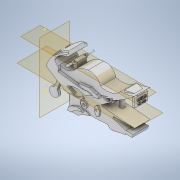
# Autodesk Inventor part: BMW S1000RR x Suzuki GXR R1000R
Saved by Autodesk Inventor 2021.1 (Build 251245000, 245)
## iProperties
Created: 2021-06-11
Part Number: BMW S1000RR x Suzuki GXR R1000R
Material: Generic
Document SubType Name: Modeling
Designer: as000166
Density: 1 g/cm^3
Appearance: Default
Author: as000166
Autodesk Inventor part; units mm, degrees
ref_plane "XY Plane" through (0, 0, 0) normal (0, 0, 1) x (1, 0, 0)
sketch "Sketch1" plane through (0, 0, 0) normal (0, 0, 1) x (1, 0, 0)
  point P0 (0, 0)
sketch "Sketch2" plane through (0, 0, 0) normal (0, 0, 1) x (1, 0, 0)
  line L0 (0, 119) -> (158.75, 119) construction
  line L1 (158.75, 119) -> (158.75, -0.0625) construction
  line L2 (158.75, -0.0625) -> (0, -0.0625) construction
  line L3 (0, -0.0625) -> (0, 119) construction
  arc A0 (51, 81) -> (25, 53) centre (68.8378, 38.3649) ccw
  arc A1 (25, 53) -> (53, 36) centre (68.2455, 92.669) ccw
  line L4 (53, 36) -> (61, 39)
  line L5 (61, 39) -> (51, 44)
  arc A2 (66, 47) -> (51, 44) centre (60.5, 35.5) ccw
  line L6 (66, 47) -> (75, 45)
  line L7 (51, 81) -> (52, 76)
  arc A3 (52, 76) -> (36, 65) centre (52.6429, 57.9286) ccw
  arc A4 (36, 65) -> (40, 60) centre (39.5, 63.7) ccw
  arc A5 (92, 62) -> (76, 72) centre (78.5, 58.2) ccw
  arc A6 (76, 72) -> (58, 63) centre (79.5, 42.5) ccw
  arc A7 (108.4973, 56.8115) -> (75, 45) centre (147.6347, -107.5867) ccw
  line L8 (108.4973, 56.8115) -> (107, 53.7361)
  arc A8 (107, 53.7361) -> (136, 72.8296) centre (44.0369, 180.937) ccw
  arc A9 (92, 62) -> (118, 69) centre (99.75, 85) ccw
  arc A10 (118, 69) -> (136, 72.8296) centre (117.9208, 113.5891) ccw
  arc A11 (40, 60) -> (58, 63) centre (47, 73.5) ccw
  point P0 (0, 0)
  constraints: 24 point on circle, 12 centre point, 10 end point, 2 other
extrude "Extrusion1" add sketch "Sketch2" along normal blind 20
sketch "Sketch3" plane through (0, 0, 20) normal (0, 0, 1) x (1, 0, 0)
  line L0 (0, 119) -> (158.75, 119) construction
  line L1 (158.75, 119) -> (158.75, -0.0625) construction
  line L2 (158.75, -0.0625) -> (0, -0.0625) construction
  line L3 (0, -0.0625) -> (0, 119) construction
  line L4 (53, 36) -> (61, 39) projected
  line L5 (55.6667, 37) -> (61, 35)
  arc A0 (61, 35) -> (69, 40) centre (60.0129, 45.4793) ccw
  arc A1 (72, 38) -> (69, 40) centre (69.1633, 36.9949) ccw
  arc A2 (72, 38) -> (75, 26) centre (73.8333, 32.0833) ccw
  arc A3 (51, 16) -> (53, 36) centre (9.8249, 30.2175) ccw
  line L6 (51, 16) -> (64, 16)
  arc A4 (79.375, 23) -> (64, 16) centre (91.4148, -23.8295) ccw
  line L7 (75, 26) -> (79.375, 23)
  point P0 (0, 0)
  constraints: 10 point on circle, 6 end point, 5 centre point, 1 point on line, 2 other
extrude "Extrusion2" add sketch "Sketch3" against normal blind 20
sketch "Sketch4" plane through (0, 0, 20) normal (0, 0, 1) x (1, 0, 0)
  line L0 (0.3227, 119.0807) -> (159.0727, 119.0807) construction
  line L1 (159.0727, 119.0807) -> (159.0727, 0.0182) construction
  line L2 (159.0727, 0.0182) -> (0.3227, 0.0182) construction
  line L3 (0.3227, 0.0182) -> (0.3227, 119.0807) construction
  line L4 (61, 39) -> (51, 44) projected
  line L5 (61, 39) -> (51.7187, 43.6406)
  arc A0 (74, 45) -> (51.7187, 43.6406) centre (64.1037, 23.9241) ccw
  arc A1 (88, 49) -> (74, 45) centre (89.4856, 17.3005) ccw
  line L6 (61, 39) -> (56.3594, 36.7402)
  line L7 (61, 35) -> (55.6667, 37) projected
  line L8 (56.3594, 36.7402) -> (61, 35)
  arc A2 (61, 35) -> (69, 40) centre (60.0129, 45.4793) ccw projected
  arc A3 (72, 38) -> (69, 40) centre (69.1633, 36.9949) ccw projected
  arc A4 (61, 35) -> (69, 40) centre (60.0129, 45.4793) ccw
  arc A5 (72, 38) -> (75, 26) centre (73.8333, 32.0833) ccw projected
  arc A6 (72, 38) -> (75, 26) centre (73.8333, 32.0833) ccw
  line L9 (75, 26) -> (79.6977, 23)
  arc A7 (109, 57) -> (88, 49) centre (124.1404, -14.3059) ccw
  line L10 (95, 51) -> (104.2405, 54.3798)
  line L11 (104.2405, 54.3798) -> (104.2405, 51)
  line L12 (104.2405, 51) -> (100.8487, 49.3312)
  line L13 (100.8487, 49.3312) -> (95, 51)
  line L14 (109, 57) -> (109, 56)
  line L15 (109, 56) -> (105, 55)
  line L16 (105, 55) -> (105, 51.3737)
  line L17 (105, 51.3737) -> (108, 53.1868)
  arc A8 (108, 53.1868) -> (111, 54) centre (108.9291, 55.6997) ccw
  line L18 (111, 54) -> (108, 51)
  line L19 (108, 51) -> (106, 51)
  line L20 (106, 51) -> (93, 42)
  line L21 (93, 42) -> (94, 40.5556)
  line L22 (94, 40.5556) -> (136, 36.9949)
  line L23 (136, 36.9949) -> (109, 36.7402)
  line L24 (109, 36.7402) -> (108, 34.2222)
  line L25 (108, 34.2222) -> (124.8199, 29)
  line L26 (124.8199, 29) -> (134, 29.0866)
  line L27 (134, 29.0866) -> (132.7312, 25)
  line L28 (132.7312, 25) -> (124.0566, 24.9182)
  line L29 (124.0566, 24.9182) -> (123.5572, 23.6607)
  line L30 (123.5572, 23.6607) -> (121.7595, 23.6438)
  line L31 (121.7595, 23.6438) -> (108, 20.3333)
  arc A9 (101.4448, 24.2894) -> (108, 20.3333) centre (106.8628, 25.8579) ccw
  arc A10 (79.6977, 23) -> (101.4448, 24.2894) centre (82.1967, 164.8855) ccw
  point P0 (0, 0)
  point P1 (110.6288, 53.6288)
  constraints: 52 end point, 16 point on circle, 8 centre point, 4 parallel, 3 point on line, 1 collinear, 1 concentric, 1 perpendicular, 1 vertical, 2 other
extrude "Extrusion3" add sketch "Sketch4" against normal blind 20 contours L4 A0 A1 A7 L14 L15 L16 L17 A8 L18 L19 L20 L21 L22 L23 L24 L25 L26 L27 L28 L29 L30 L31 A9 A10 L9 A5 A3 A2 L7 L6
sketch "Sketch5" plane through (0, 0, 20) normal (0, 0, 1) x (1, 0, 0)
  line L0 (0, 119) -> (158.75, 119) construction
  line L1 (158.75, 119) -> (158.75, -0.0625) construction
  line L2 (158.75, -0.0625) -> (0, -0.0625) construction
  line L3 (0, -0.0625) -> (0, 119) construction
  arc A0 (25, 53) -> (53, 36) centre (68.2455, 92.669) ccw projected
  line L4 (38.4827, 42.0925) -> (38.4827, 42.0925)
  line L5 (36.9918, 43) -> (32.2278, 31.5476)
  line L6 (40.4226, 41) -> (36, 30)
  arc A1 (32.2278, 31.5476) -> (36, 30) centre (32, 25.6214) ccw
  point P0 (0, 0)
  constraints: 6 end point, 6 point on circle, 1 centre point, 1 tangent, 2 other
extrude "Extrusion4" add sketch "Sketch5" against normal blind 20
sketch "Sketch6" plane through (0, 0, 20) normal (0, 0, 1) x (1, 0, 0)
  line L0 (0, 119) -> (158.75, 119) construction
  line L1 (158.75, 119) -> (158.75, -0.0625) construction
  line L2 (158.75, -0.0625) -> (0, -0.0625) construction
  line L3 (0, -0.0625) -> (0, 119) construction
  line L4 (52, 76) -> (51, 81) projected
  arc A0 (51, 81) -> (25, 53) centre (68.8378, 38.3649) ccw projected
  arc A1 (51.5, 78.5) -> (25, 53) centre (61.7966, 41.28) ccw
  arc A2 (51, 16) -> (53, 36) centre (9.8249, 30.2175) ccw projected
  arc A3 (25, 53) -> (53, 36) centre (128.25, 191.5) ccw
  line L5 (53, 36) -> (60.7223, 38.8959)
  line L6 (55.6667, 37) -> (61, 39) projected
  arc A4 (65.6621, 47.1556) -> (51.7187, 43.6406) centre (64.1037, 23.9241) ccw projected
  line L7 (61, 39) -> (51.7187, 43.6406)
  line L8 (51.7187, 43.6406) -> (51, 44) projected
  arc A5 (65.6621, 47.1556) -> (51.7187, 43.6406) centre (64.1037, 23.9241) ccw
  line L9 (65.6621, 47.1556) -> (75, 45)
  line L10 (75, 45) -> (84.0807, 49)
  arc A6 (101.5471, 55) -> (82, 48.1393) centre (147.6347, -107.5867) ccw projected
  line L11 (84.0807, 49) -> (77, 51)
  arc A7 (71.2365, 50) -> (77, 51) centre (72.017, 62.6105) ccw
  line L12 (71.2365, 50) -> (40, 54)
  line L13 (51.5, 78.5) -> (52, 76)
  arc A8 (52, 76) -> (36.049, 65) centre (52.301, 58.4983) ccw
  arc A9 (36.049, 65) -> (40, 60) centre (49.8238, 71.8238) ccw
  arc A10 (40, 54) -> (40, 60) centre (36, 57) ccw
  point P0 (0, 0)
  point P1 (27.4841, 59)
  constraints: 15 point on circle, 14 end point, 7 centre point, 1 collinear, 1 concentric, 1 midpoint, 1 point on line, 2 other
extrude "Extrusion5" add sketch "Sketch6" along normal blind 3 and the other way blind 23 contours A8 A9 A10 L12 A7 L11 L10 L9 A4 L7 L6 L5 A3 A0 A1 L4
sketch "Sketch7" plane through (36.9918, 43, 0) normal (-0.9233002, 0.3840791, 0) x (0, 0, 1)
  line L0 (0, -0.3147) -> (20, -0.3147) projected
  line L1 (4, -0.3147) -> (17, -0.3147)
  line L2 (17, -0.3147) -> (17, -23.8935)
  line L3 (20, -23.8935) -> (0, -23.8935) projected
  line L4 (17, -23.8935) -> (4, -23.8935)
  line L5 (4, -23.8935) -> (4, -0.3147)
  point P0 (0, -53.9097)
  constraints: 8 end point, 3 point on line, 2 perpendicular, 1 horizontal
extrude "Extrusion6" cut sketch "Sketch7" along normal blind 9 and the other way blind 9
sketch "Sketch10" plane through (0, 0, 20) normal (0, 0, 1) x (1, 0, 0)
  line L0 (0, 117) -> (158.75, 117) construction
  line L1 (158.75, 117) -> (158.75, -2.0625) construction
  line L2 (158.75, -2.0625) -> (0, -2.0625) construction
  line L3 (0, -2.0625) -> (0, 117) construction
  line L4 (66, 54) -> (81, 56)
  arc A0 (81, 56) -> (90.0213, 52.996) centre (96.5, 87.5) ccw
  arc A1 (93, 49.9999) -> (90.0213, 52.996) centre (89.3337, 49.3336) ccw
  arc A2 (66, 54) -> (75.4151, 50.8696) centre (73.5, 60.8333) ccw
  arc A3 (84.2663, 49.9712) -> (75.4151, 50.8696) centre (78.3411, 35.6463) ccw
  line L5 (84.2663, 49.9712) -> (86, 48)
  line L6 (86, 48) -> (93, 49.9999)
  point P0 (0, 0)
  constraints: 8 point on circle, 6 end point, 4 centre point, 2 tangent, 2 other
extrude "Extrusion7" add sketch "Sketch10" along normal blind 3 and the other way blind 23
ref_plane "Work Plane1" through (0, 70, 0) normal (0, 1, 0) x (-1, 0, 0)
sketch "Sketch11" plane through (0, 70, 0) normal (0, 1, 0) x (-1, 0, 0)
  line L0 (-53, 0) -> (-53, 20) projected
  line L1 (-53, 16) -> (-53, 4)
  line L2 (-53, 4) -> (-58, 4)
  line L3 (-58, 4) -> (-58, 16)
  line L4 (-58, 0) -> (-58, 20) projected
  line L5 (-53, 16) -> (-58, 16)
  point P0 (0, 0)
  dimension "d27" = 12
  dimension "d28" = 5
  constraints: 8 end point, 3 point on line, 1 perpendicular
  measures "d27" distance of L1.start L1.end
  measures "d28" distance of L1.end L2.end
extrude "Extrusion8" add sketch "Sketch11" against normal up to surface
sketch "Sketch12" plane through (0, 70, 0) normal (0, 1, 0) x (1, 0, 0)
  point P0 (0, 0)
sketch "Sketch13" plane through (0, 70, 0) normal (0, 1, 0) x (1, 0, 0)
  line L0 (53, -4) -> (53, -16) projected
  line L1 (53, -4) -> (53, -16)
  line L2 (53, -16) -> (60.2469, -16) construction
  line L3 (58, -16) -> (58, -20) projected
  line L4 (58, -16) -> (58, -4)
  line L5 (58, -4) -> (58, -16)
  line L6 (58, 0) -> (58, -4) projected
  line L7 (58, -4) -> (58, -16)
  line L8 (53, -16) -> (54, -20)
  line L9 (54, -20) -> (56, -20)
  line L10 (58, -20) -> (40, -20) projected
  line L11 (58, -16) -> (56, -20)
  line L12 (53, -4) -> (54, 0)
  line L13 (58, 0) -> (40, 0) projected
  line L14 (54, 0) -> (56, 0)
  line L15 (58, -4) -> (56, 0)
  line L16 (54, -16) -> (57, -16)
  line L17 (57, -16) -> (56, -18)
  line L18 (56, -18) -> (54.5, -18)
  line L19 (54.5, -18) -> (54, -16)
  line L20 (54, -4) -> (56.8824, -4)
  line L21 (56, -2) -> (54.5, -2)
  line L22 (54.5, -2) -> (54, -4)
  line L23 (56.8824, -4) -> (56, -2)
  point P0 (0, 0)
  dimension "d31" = 12
  dimension "d35" = 1.5
  dimension "d36" = 1.5
  constraints: 38 end point, 5 point on line, 3 collinear, 2 horizontal, 1 parallel, 1 vertical
  measures "d31" distance of L0.start L0.end
  measures "d35" distance of L17.end L18.end
  measures "d36" distance of L21.start L21.end
extrude "Extrusion9" add sketch "Sketch13" against normal blind 2 contours L12 L13 L15 L4 L11 L9 L8 L0
sketch "Sketch14" plane through (54, 70, 20) normal (0, 0, 1) x (1, 0, 0)
  circle A0 centre (1, -1) radius 1
  point P0 (-54, -70)
  constraints: 1 centre point
extrude "Extrusion10" add sketch "Sketch14" along normal blind 7
sketch "Sketch15" plane through (56, 70, 0) normal (0, 0, -1) x (-1, 0, 0)
  circle A0 centre (1, -1) radius 1
  line L0 (2, 0) -> (2, -1) projected
  point P0 (56, -70)
  constraints: 1 horizontal alignment, 1 vertical, 1 other
extrude "Extrusion11" add sketch "Sketch15" along normal blind 8
sketch "Sketch16" plane through (0, 70, 0) normal (0, 1, 0) x (-1, 0, 0)
  line L0 (-121, 18) -> (-121, 2)
  line L1 (-121, 2) -> (-134, 5.4833)
  line L2 (-134, 20) -> (-134, 0) projected
  line L3 (-121, 18) -> (-108.0418, 18) construction
  line L4 (-121, 18) -> (-134, 14.5167)
  line L5 (-121, 18) -> (-107.5414, 18) construction
  line L6 (-134, 14.5167) -> (-134, 5.4833)
  point P0 (0, 0)
  dimension "d43" = 75
  dimension "d45" = 165
  constraints: 12 end point, 2 horizontal, 2 point on line, 1 collinear, 1 equal length, 1 vertical
  measures "d43" angle of L0 L1
  measures "d45" angle of L4 L5
extrude "Extrusion12" add sketch "Sketch16" along normal blind 1 and the other way blind 0.95
sketch "Sketch17" plane through (134, 69.05, 5.4833) normal (1, 0, 0) x (0, 0, -1)
  line L0 (3.4833, 1.95) -> (-12.5167, 1.95) projected
  line L1 (-9, 1.95) -> (0, 1.95)
  line L2 (0, 1.95) -> (0, -0.05)
  line L3 (5.4833, -0.05) -> (-14.5167, -0.05) projected
  line L4 (0, -0.05) -> (4, -0.05)
  line L5 (-9.0333, 0) -> (-9.0333, 1.95) projected
  line L6 (-9.0333, 0) -> (-13.0333, 0)
  line L7 (-13.0333, 0) -> (-13.0333, -5)
  line L8 (-13.0333, -5) -> (-13.0333, -11)
  line L9 (4, -0.05) -> (4, -11)
  line L10 (-13.0333, -11) -> (4, -11)
  point P0 (5.4833, -69.05)
  point P1 (-13.0333, -0.05)
  dimension "d51" = 4
  dimension "d52" = 5
  dimension "d75" = 6
  constraints: 16 end point, 3 point on line, 2 perpendicular, 1 horizontal, 1 vertical
  measures "d51" distance of L5.start L6.end
  measures "d52" distance of L6.end L7.end
  measures "d75" distance of L7.end L8.end
extrude "Extrusion13" add sketch "Sketch17" along normal blind 0.75 and the other way blind 2 contours L3 L9 L10 L8 L7
sketch "Sketch18" plane through (0, 0, 20) normal (0, 0, 1) x (1, 0, 0)
  line L0 (0, 118) -> (158.75, 118) construction
  line L1 (158.75, 118) -> (158.75, -1.0625) construction
  line L2 (158.75, -1.0625) -> (0, -1.0625) construction
  line L3 (0, -1.0625) -> (0, 118) construction
  arc A0 (72, 24) -> (57, 17) centre (72.2778, 3.8333) ccw
  line L4 (57, 17) -> (52, 17)
  arc A1 (59, 25) -> (52, 17) centre (65.1, 12.6) ccw
  line L5 (59, 25) -> (65, 27)
  arc A2 (72, 24) -> (65, 27) centre (64.5774, 16.3472) ccw
  point P0 (0, 0)
  constraints: 6 point on circle, 4 end point, 3 centre point, 2 other
extrude "Extrusion14" add sketch "Sketch18" along normal blind 3 and the other way blind 23
sketch "Sketch19" plane through (0, 0, 20) normal (0, 0, 1) x (1, 0, 0)
  line L0 (0, 119) -> (158.75, 119) construction
  line L1 (158.75, 119) -> (158.75, -0.0625) construction
  line L2 (158.75, -0.0625) -> (0, -0.0625) construction
  line L3 (0, -0.0625) -> (0, 119) construction
  circle A0 centre (72, 32) radius 4
  circle A1 centre (72, 32) radius 1.7911
  point P0 (0, 0)
  constraints: 2 centre point, 1 coincident, 2 other
extrude "Extrusion15" add sketch "Sketch19" along normal blind 1.5 and the other way blind 21.5
sketch "Sketch20" plane through (0, 0, 20) normal (0, 0, 1) x (1, 0, 0)
  line L0 (0, 119) -> (158.75, 119) construction
  line L1 (158.75, 119) -> (158.75, -0.0625) construction
  line L2 (158.75, -0.0625) -> (0, -0.0625) construction
  line L3 (0, -0.0625) -> (0, 119) construction
  line L4 (87, 38) -> (90, 40)
  arc A0 (91, 28) -> (90, 40) centre (79.25, 33.0625) ccw
  arc A1 (87, 38) -> (88.5, 26.8549) centre (95.5979, 33.4837) ccw
  line L5 (88.5, 26.8549) -> (91, 28)
  circle A2 centre (88, 34) radius 1
  point P0 (0, 0)
  constraints: 4 end point, 4 point on circle, 3 centre point, 2 other
extrude "Extrusion16" add sketch "Sketch20" along normal blind 1.5 and the other way blind 21.5
sketch "Sketch21" plane through (134.75, 69.05, 5.4833) normal (1, 0, 0) x (0, 0, -1)
  line L0 (-10.1051, -1.0894) -> (0.9281, -1.0894) construction
  line L1 (0.9281, -1.0894) -> (0.9281, -4.0805) construction
  line L2 (0.9281, -4.0805) -> (-10.1051, -4.0805) construction
  line L3 (-10.1051, -4.0805) -> (-10.1051, -1.0894) construction
  line L4 (-8.5838, -2.0986) -> (-7.0277, -2.0986)
  line L5 (-7.0277, -2.0986) -> (-7.0277, -5.0947)
  line L6 (-7.0277, -5.0947) -> (-7.3562, -5.0947)
  line L7 (-7.3562, -5.0947) -> (-7.3562, -4.8823)
  line L8 (-7.3562, -4.8823) -> (-8.2553, -4.8823)
  line L9 (-8.2553, -4.8823) -> (-8.2553, -5.1935)
  line L10 (-8.2553, -5.1935) -> (-8.5838, -5.1935)
  line L11 (-8.5838, -5.1935) -> (-8.5838, -2.0986)
  line L12 (-10.582, -2.968) -> (-10.582, -2.6568)
  line L13 (-10.582, -2.6568) -> (-9.8114, -2.6568)
  line L14 (-9.8114, -2.6568) -> (-9.8114, -2.148)
  spline S0 degree 2 poles (-9.8114, -2.148) (-10.2214, -2.2146) (-10.4511, -2.2295) knots 0 0 0 1 1 1
  line L15 (-10.4511, -2.2295) -> (-10.582, -1.9355)
  spline S1 degree 2 poles (-10.582, -1.9355) (-9.7472, -1.854) (-9.0901, -1.607) knots 0 0 0 1 1 1
  line L16 (-9.0901, -1.607) -> (-8.895, -1.9034)
  spline S2 degree 2 poles (-8.895, -1.9034) (-8.8777, -2.017) (-8.9938, -1.9528) knots 0 0 0 1 1 1
  line L17 (-8.9938, -1.9528) -> (-9.4853, -2.0837)
  line L18 (-9.4853, -2.0837) -> (-9.4853, -2.6568)
  line L19 (-9.4853, -2.6568) -> (-8.7468, -2.6568)
  line L20 (-8.7468, -2.6568) -> (-8.7468, -2.968)
  line L21 (-8.7468, -2.968) -> (-9.4853, -2.968)
  line L22 (-9.4853, -2.968) -> (-9.4853, -3.3113)
  spline S3 degree 2 poles (-9.4853, -3.3113) (-8.9938, -3.5238) (-8.732, -3.835) knots 0 0 0 1 1 1
  line L23 (-8.732, -3.835) -> (-8.9444, -4.1462)
  spline S4 degree 2 poles (-8.9444, -4.1462) (-9.2383, -3.8177) (-9.4853, -3.6547) knots 0 0 0 1 1 1
  line L24 (-9.4853, -3.6547) -> (-9.4853, -5.275)
  line L25 (-9.4853, -5.275) -> (-9.8114, -5.275)
  line L26 (-9.8114, -5.275) -> (-9.8114, -3.7041)
  spline S5 degree 2 poles (-9.8114, -3.7041) (-10.0584, -4.1956) (-10.4338, -4.571) knots 0 0 0 1 1 1
  line L27 (-10.4338, -4.571) -> (-10.6783, -4.2771)
  spline S6 degree 2 poles (-10.6783, -4.2771) (-10.0732, -3.7041) (-9.8287, -2.968) knots 0 0 0 1 1 1
  line L28 (-9.8287, -2.968) -> (-10.582, -2.968)
  line L29 (-8.2553, -2.4098) -> (-8.2553, -4.571)
  line L30 (-8.2553, -4.571) -> (-7.3562, -4.571)
  line L31 (-7.3562, -4.571) -> (-7.3562, -2.4098)
  line L32 (-7.3562, -2.4098) -> (-8.2553, -2.4098)
  spline S7 degree 2 poles (-3.6882, -4.0474) (-3.8833, -4.7341) (-4.5058, -5.275) knots 0 0 0 1 1 1
  line L33 (-4.5058, -5.275) -> (-4.7207, -4.9638)
  spline S8 degree 2 poles (-4.7207, -4.9638) (-3.8833, -4.3265) (-3.8833, -3.3928) knots 0 0 0 1 1 1
  line L34 (-3.8833, -3.3928) -> (-3.8833, -2.558)
  line L35 (-3.8833, -2.558) -> (-4.0315, -2.558)
  spline S9 degree 2 poles (-4.0315, -2.558) (-4.0982, -2.8025) (-4.3255, -3.2125) knots 0 0 0 1 1 1
  line L36 (-4.3255, -3.2125) -> (-4.6046, -3.0643)
  spline S10 degree 2 poles (-4.6046, -3.0643) (-4.2291, -2.5259) (-4.1303, -1.5922) knots 0 0 0 1 1 1
  line L37 (-4.1303, -1.5922) -> (-3.8191, -1.6416)
  spline S11 degree 2 poles (-3.8191, -1.6416) (-3.7203, -1.6564) (-3.8364, -1.7379) knots 0 0 0 1 1 1
  spline S12 degree 2 poles (-3.8364, -1.7379) (-3.9327, -2.1652) (-3.9673, -2.2962) knots 0 0 0 1 1 1
  line L38 (-3.9673, -2.2962) -> (-3.0658, -2.2962)
  line L39 (-3.0658, -2.2962) -> (-3.0336, -2.2146)
  line L40 (-3.0336, -2.2146) -> (-2.7224, -2.4098)
  spline S13 degree 2 poles (-2.7224, -2.4098) (-2.673, -2.4419) (-2.7545, -2.4913) knots 0 0 0 1 1 1
  spline S14 degree 2 poles (-2.7545, -2.4913) (-2.8854, -3.0816) (-3.1152, -3.541) knots 0 0 0 1 1 1
  line L41 (-3.1152, -3.541) -> (-3.3943, -3.425)
  spline S15 degree 2 poles (-3.3943, -3.425) (-3.1646, -2.968) (-3.083, -2.558) knots 0 0 0 1 1 1
  line L42 (-3.083, -2.558) -> (-3.5573, -2.558)
  line L43 (-3.5573, -2.558) -> (-3.5573, -3.3434)
  spline S16 degree 2 poles (-3.5573, -3.3434) (-3.5573, -4.2771) (-2.7051, -4.9317) knots 0 0 0 1 1 1
  line L44 (-2.7051, -4.9317) -> (-2.9521, -5.2108)
  spline S17 degree 2 poles (-2.9521, -5.2108) (-3.5252, -4.6871) (-3.6882, -4.0474) knots 0 0 0 1 1 1
  spline S18 degree 2 poles (-4.7528, -5.0132) (-4.7528, -5.2602) (-4.9973, -5.2602) knots 0 0 0 1 1 1
  line L45 (-4.9973, -5.2602) -> (-5.4073, -5.2602)
  line L46 (-5.4073, -5.2602) -> (-5.4567, -4.949)
  line L47 (-5.4567, -4.949) -> (-5.0961, -4.949)
  spline S19 degree 2 poles (-5.0961, -4.949) (-5.0294, -4.949) (-5.0294, -4.8823) knots 0 0 0 1 1 1
  line L48 (-5.0294, -4.8823) -> (-5.0294, -3.7041)
  line L49 (-5.0294, -3.7041) -> (-6.4719, -3.7041)
  line L50 (-6.4719, -3.7041) -> (-6.4719, -3.3928)
  line L51 (-6.4719, -3.3928) -> (-4.4416, -3.3928)
  line L52 (-4.4416, -3.3928) -> (-4.4416, -3.7041)
  line L53 (-4.4416, -3.7041) -> (-4.7528, -3.7041)
  line L54 (-4.7528, -3.7041) -> (-4.7528, -5.0132)
  spline S20 degree 2 poles (-4.7528, -3.0149) (-4.7528, -3.2768) (-4.9652, -3.2768) knots 0 0 0 1 1 1
  line L55 (-4.9652, -3.2768) -> (-5.2443, -3.2768)
  line L56 (-5.2443, -3.2768) -> (-5.2764, -3.0149)
  line L57 (-5.2764, -3.0149) -> (-5.0961, -3.0149)
  spline S21 degree 2 poles (-5.0961, -3.0149) (-5.0294, -3.0149) (-5.0294, -2.9507) knots 0 0 0 1 1 1
  line L58 (-5.0294, -2.9507) -> (-5.0294, -2.017)
  line L59 (-5.0294, -2.017) -> (-6.3558, -2.017)
  line L60 (-6.3558, -2.017) -> (-6.3558, -1.7058)
  line L61 (-6.3558, -1.7058) -> (-4.4564, -1.7058)
  line L62 (-4.4564, -1.7058) -> (-4.4564, -2.017)
  line L63 (-4.4564, -2.017) -> (-4.7528, -2.017)
  line L64 (-4.7528, -2.017) -> (-4.7528, -3.0149)
  line L65 (-5.2937, -3.8992) -> (-5.2937, -4.702)
  line L66 (-5.2937, -4.702) -> (-5.9804, -4.702)
  line L67 (-5.9804, -4.702) -> (-5.9804, -4.8823)
  line L68 (-5.9804, -4.8823) -> (-6.2101, -4.8823)
  line L69 (-6.2101, -4.8823) -> (-6.2101, -3.8992)
  line L70 (-6.2101, -3.8992) -> (-5.2937, -3.8992)
  line L71 (-5.3085, -2.2146) -> (-5.3085, -2.9507)
  line L72 (-5.3085, -2.9507) -> (-5.931, -2.9507)
  line L73 (-5.931, -2.9507) -> (-5.931, -3.0989)
  line L74 (-5.931, -3.0989) -> (-6.1607, -3.0989)
  line L75 (-6.1607, -3.0989) -> (-6.1607, -2.2146)
  line L76 (-6.1607, -2.2146) -> (-5.3085, -2.2146)
  line L77 (-5.521, -4.0968) -> (-5.9804, -4.0968)
  line L78 (-5.9804, -4.0968) -> (-5.9804, -4.5068)
  line L79 (-5.9804, -4.5068) -> (-5.521, -4.5068)
  line L80 (-5.521, -4.5068) -> (-5.521, -4.0968)
  line L81 (-5.5382, -2.4098) -> (-5.931, -2.4098)
  line L82 (-5.931, -2.4098) -> (-5.931, -2.7531)
  line L83 (-5.931, -2.7531) -> (-5.5382, -2.7531)
  line L84 (-5.5382, -2.7531) -> (-5.5382, -2.4098)
  spline S22 degree 2 poles (1.2247, -2.3604) (1.3877, -2.395) (1.2395, -2.4913) knots 0 0 0 1 1 1
  line L85 (1.2395, -2.4913) -> (1.2395, -5.112)
  line L86 (1.2395, -5.112) -> (0.864, -5.112)
  line L87 (0.864, -5.112) -> (0.864, -4.8502)
  line L88 (0.864, -4.8502) -> (-1.6406, -4.8502)
  line L89 (-1.6406, -4.8502) -> (-1.6406, -5.1762)
  line L90 (-1.6406, -5.1762) -> (-2.0185, -5.1762)
  line L91 (-2.0185, -5.1762) -> (-2.0185, -2.3604)
  line L92 (-2.0185, -2.3604) -> (-1.6578, -2.3604)
  spline S23 degree 2 poles (-1.6578, -2.3604) (-1.4948, -2.395) (-1.6406, -2.4913) knots 0 0 0 1 1 1
  line L93 (-1.6406, -2.4913) -> (-1.6406, -4.4895)
  line L94 (-1.6406, -4.4895) -> (-0.5933, -4.4895)
  line L95 (-0.5933, -4.4895) -> (-0.5933, -1.6737)
  line L96 (-0.5933, -1.6737) -> (-0.2326, -1.6737)
  spline S24 degree 2 poles (-0.2326, -1.6737) (-0.0696, -1.7058) (-0.2178, -1.8046) knots 0 0 0 1 1 1
  line L97 (-0.2178, -1.8046) -> (-0.2178, -4.4895)
  line L98 (-0.2178, -4.4895) -> (0.864, -4.4895)
  line L99 (0.864, -4.4895) -> (0.864, -2.3604)
  line L100 (0.864, -2.3604) -> (1.2247, -2.3604)
  line L101 (-7.7403, -8.9028) -> (-8.1034, -8.9028)
  line L102 (-8.1034, -8.9028) -> (-8.1034, -9.9501)
  line L103 (-8.1034, -9.9501) -> (-8.4961, -9.9501)
  line L104 (-8.4961, -9.9501) -> (-8.4961, -8.9028)
  line L105 (-8.4961, -8.9028) -> (-9.8422, -8.9028)
  line L106 (-9.8422, -8.9028) -> (-9.8422, -8.473)
  line L107 (-9.8422, -8.473) -> (-8.4788, -6.9021)
  line L108 (-8.4788, -6.9021) -> (-8.1034, -6.9021)
  line L109 (-8.1034, -6.9021) -> (-8.1034, -8.5743)
  line L110 (-8.1034, -8.5743) -> (-7.7403, -8.5743)
  line L111 (-7.7403, -8.5743) -> (-7.7403, -8.9028)
  line L112 (-8.4961, -8.5743) -> (-8.4961, -7.3838)
  line L113 (-8.4961, -7.3838) -> (-9.5211, -8.5743)
  line L114 (-9.5211, -8.5743) -> (-8.4961, -8.5743)
  line L115 (-5.5345, -9.9501) -> (-7.4142, -9.9501)
  line L116 (-7.4142, -9.9501) -> (-7.4142, -9.5179)
  spline S25 degree 2 poles (-7.4142, -9.5179) (-7.2117, -9.3277) (-6.8511, -8.9745) (-6.6782, -8.7843) knots 0 0 0 1 2 2 2
  spline S26 degree 2 poles (-6.6782, -8.7843) (-6.3299, -8.4014) (-6.0755, -7.942) (-6.0755, -7.6975) knots 0 0 0 1 2 2 2
  spline S27 degree 2 poles (-6.0755, -7.6975) (-6.0755, -7.569) (-6.1545, -7.3764) (-6.2261, -7.3146) knots 0 0 0 1 2 2 2
  spline S28 degree 2 poles (-6.2261, -7.3146) (-6.2978, -7.2529) (-6.4855, -7.1911) (-6.5991, -7.1911) knots 0 0 0 1 2 2 2
  spline S29 degree 2 poles (-6.5991, -7.1911) (-6.7078, -7.1911) (-6.9301, -7.2455) (-7.0314, -7.2874) knots 0 0 0 1 2 2 2
  spline S30 degree 2 poles (-7.0314, -7.2874) (-7.1178, -7.322) (-7.2784, -7.4208) (-7.3278, -7.4554) knots 0 0 0 1 2 2 2
  line L117 (-7.3278, -7.4554) -> (-7.35, -7.4554)
  line L118 (-7.35, -7.4554) -> (-7.35, -7.0207)
  spline S31 degree 2 poles (-7.35, -7.0207) (-7.224, -6.9589) (-6.772, -6.8379) (-6.5695, -6.8379) knots 0 0 0 1 2 2 2
  spline S32 degree 2 poles (-6.5695, -6.8379) (-6.1422, -6.8379) (-5.6605, -7.2899) (-5.6605, -7.6752) knots 0 0 0 1 2 2 2
  spline S33 degree 2 poles (-5.6605, -7.6752) (-5.6605, -7.8555) (-5.7445, -8.1569) (-5.8186, -8.2853) knots 0 0 0 1 2 2 2
  spline S34 degree 2 poles (-5.8186, -8.2853) (-5.8927, -8.4187) (-6.1076, -8.6805) (-6.2261, -8.8065) knots 0 0 0 1 2 2 2
  spline S35 degree 2 poles (-6.2261, -8.8065) (-6.4188, -9.0165) (-6.8906, -9.466) (-7.0314, -9.5969) knots 0 0 0 1 2 2 2
  line L119 (-7.0314, -9.5969) -> (-5.5345, -9.5969)
  line L120 (-5.5345, -9.5969) -> (-5.5345, -9.9501)
  line L121 (-4.0105, -8.8016) -> (-5.164, -8.8016)
  line L122 (-5.164, -8.8016) -> (-5.164, -8.4311)
  line L123 (-5.164, -8.4311) -> (-4.0105, -8.4311)
  line L124 (-4.0105, -8.4311) -> (-4.0105, -8.8016)
  spline S36 degree 2 poles (-1.6788, -8.9621) (-1.6788, -9.1968) (-1.8345, -9.5944) (-1.9654, -9.7278) knots 0 0 0 1 2 2 2
  spline S37 degree 2 poles (-1.9654, -9.7278) (-2.1012, -9.8686) (-2.4421, -10.0143) (-2.6471, -10.0143) knots 0 0 0 1 2 2 2
  spline S38 degree 2 poles (-2.6471, -10.0143) (-2.8521, -10.0143) (-3.1905, -9.876) (-3.3189, -9.7377) knots 0 0 0 1 2 2 2
  spline S39 degree 2 poles (-3.3189, -9.7377) (-3.477, -9.5722) (-3.6549, -9.0165) (-3.6549, -8.6114) knots 0 0 0 1 2 2 2
  spline S40 degree 2 poles (-3.6549, -8.6114) (-3.6549, -8.2137) (-3.4918, -7.574) (-3.3214, -7.3368) knots 0 0 0 1 2 2 2
  spline S41 degree 2 poles (-3.3214, -7.3368) (-3.1559, -7.1047) (-2.6323, -6.8453) (-2.2889, -6.8453) knots 0 0 0 1 2 2 2
  spline S42 degree 2 poles (-2.2889, -6.8453) (-2.1877, -6.8453) (-2.0098, -6.8651) (-1.9431, -6.8873) knots 0 0 0 1 2 2 2
  line L125 (-1.9431, -6.8873) -> (-1.9431, -7.28)
  line L126 (-1.9431, -7.28) -> (-1.9604, -7.28)
  spline S43 degree 2 poles (-1.9604, -7.28) (-2.0172, -7.2504) (-2.2247, -7.1985) (-2.3433, -7.1985) knots 0 0 0 1 2 2 2
  spline S44 degree 2 poles (-2.3433, -7.1985) (-2.7237, -7.1985) (-3.1905, -7.7123) (-3.235, -8.2162) knots 0 0 0 1 2 2 2
  spline S45 degree 2 poles (-3.235, -8.2162) (-3.0892, -8.1149) (-2.7829, -8.0037) (-2.6002, -8.0037) knots 0 0 0 1 2 2 2
  spline S46 degree 2 poles (-2.6002, -8.0037) (-2.4223, -8.0037) (-2.1556, -8.0754) (-2.0098, -8.1841) knots 0 0 0 1 2 2 2
  spline S47 degree 2 poles (-2.0098, -8.1841) (-1.8419, -8.31) (-1.6788, -8.7003) (-1.6788, -8.9621) knots 0 0 0 1 2 2 2
  spline S48 degree 2 poles (-2.0938, -8.9794) (-2.0938, -8.7917) (-2.1926, -8.5373) (-2.3013, -8.4483) knots 0 0 0 1 2 2 2
  spline S49 degree 2 poles (-2.3013, -8.4483) (-2.3828, -8.3841) (-2.5853, -8.3421) (-2.6915, -8.3421) knots 0 0 0 1 2 2 2
  spline S50 degree 2 poles (-2.6915, -8.3421) (-2.8348, -8.3421) (-3.104, -8.4286) (-3.235, -8.5101) knots 0 0 0 1 2 2 2
  spline S51 degree 2 poles (-3.235, -8.5101) (-3.2374, -8.5546) (-3.2424, -8.6385) (-3.2424, -8.7028) knots 0 0 0 1 2 2 2
  spline S52 degree 2 poles (-3.2424, -8.7028) (-3.2424, -9.0189) (-3.1189, -9.4067) (-3.025, -9.508) knots 0 0 0 1 2 2 2
  spline S53 degree 2 poles (-3.025, -9.508) (-2.9386, -9.6043) (-2.7508, -9.6809) (-2.6446, -9.6809) knots 0 0 0 1 2 2 2
  spline S54 degree 2 poles (-2.6446, -9.6809) (-2.3976, -9.6809) (-2.0938, -9.3301) (-2.0938, -8.9794) knots 0 0 0 1 2 2 2
  spline S55 degree 2 poles (-1.4022, -7.8926) (-1.4022, -7.6579) (-1.2491, -7.2677) (-1.1157, -7.1269) knots 0 0 0 1 2 2 2
  spline S56 degree 2 poles (-1.1157, -7.1269) (-0.9897, -6.991) (-0.6217, -6.8404) (-0.434, -6.8404) knots 0 0 0 1 2 2 2
  spline S57 degree 2 poles (-0.434, -6.8404) (-0.224, -6.8404) (0.1169, -6.9812) (0.2428, -7.1145) knots 0 0 0 1 2 2 2
  spline S58 degree 2 poles (0.2428, -7.1145) (0.4009, -7.2825) (0.5738, -7.8259) (0.5738, -8.2433) knots 0 0 0 1 2 2 2
  spline S59 degree 2 poles (0.5738, -8.2433) (0.5738, -8.6212) (0.4034, -9.298) (0.2379, -9.5228) knots 0 0 0 1 2 2 2
  spline S60 degree 2 poles (0.2379, -9.5228) (0.0625, -9.7599) (-0.4315, -10.0094) (-0.7921, -10.0094) knots 0 0 0 1 2 2 2
  spline S61 degree 2 poles (-0.7921, -10.0094) (-0.8736, -10.0094) (-1.0589, -9.9921) (-1.1379, -9.9674) knots 0 0 0 1 2 2 2
  line L127 (-1.1379, -9.9674) -> (-1.1379, -9.5747)
  line L128 (-1.1379, -9.5747) -> (-1.1181, -9.5747)
  spline S62 degree 2 poles (-1.1181, -9.5747) (-1.0663, -9.6043) (-0.8489, -9.6562) (-0.7378, -9.6562) knots 0 0 0 1 2 2 2
  spline S63 degree 2 poles (-0.7378, -9.6562) (-0.3376, -9.6562) (0.1193, -9.1276) (0.1514, -8.6385) knots 0 0 0 1 2 2 2
  spline S64 degree 2 poles (0.1514, -8.6385) (-0.0116, -8.7497) (-0.308, -8.851) (-0.4834, -8.851) knots 0 0 0 1 2 2 2
  spline S65 degree 2 poles (-0.4834, -8.851) (-0.6513, -8.851) (-0.9304, -8.7769) (-1.0712, -8.6707) knots 0 0 0 1 2 2 2
  spline S66 degree 2 poles (-1.0712, -8.6707) (-1.2342, -8.5447) (-1.4022, -8.1618) (-1.4022, -7.8926) knots 0 0 0 1 2 2 2
  spline S67 degree 2 poles (0.1613, -8.1519) (0.1613, -7.8432) (0.0477, -7.4529) (-0.0536, -7.3467) knots 0 0 0 1 2 2 2
  spline S68 degree 2 poles (-0.0536, -7.3467) (-0.1425, -7.2479) (-0.3277, -7.1738) (-0.4364, -7.1738) knots 0 0 0 1 2 2 2
  spline S69 degree 2 poles (-0.4364, -7.1738) (-0.6884, -7.1738) (-0.9872, -7.5344) (-0.9872, -7.8753) knots 0 0 0 1 2 2 2
  spline S70 degree 2 poles (-0.9872, -7.8753) (-0.9872, -8.068) (-0.8884, -8.3174) (-0.7798, -8.4064) knots 0 0 0 1 2 2 2
  spline S71 degree 2 poles (-0.7798, -8.4064) (-0.7007, -8.4706) (-0.5056, -8.5126) (-0.392, -8.5126) knots 0 0 0 1 2 2 2
  spline S72 degree 2 poles (-0.392, -8.5126) (-0.2611, -8.5126) (0.0403, -8.4212) (0.1539, -8.3446) knots 0 0 0 1 2 2 2
  spline S73 degree 2 poles (0.1539, -8.3446) (0.1564, -8.315) (0.1613, -8.2137) (0.1613, -8.1519) knots 0 0 0 1 2 2 2
  point P0 (5.4833, -69.05)
  constraints: 2 other
extrude "Extrusion17" add sketch "Sketch21" along normal blind 1
sketch "Sketch22" plane through (0, 69.05, 0) normal (0, -1, 0) x (1, 0, 0)
  point P0 (0, 0)
sketch "Sketch23" plane through (0, 0, 20) normal (0, 0, 1) x (1, 0, 0)
  line L0 (0, 119) -> (158.75, 119) construction
  line L1 (158.75, 119) -> (158.75, -0.0625) construction
  line L2 (158.75, -0.0625) -> (0, -0.0625) construction
  line L3 (0, -0.0625) -> (0, 119) construction
  arc A0 (51, 16) -> (53, 36) centre (9.8249, 30.2175) ccw projected
  line L4 (51, 16) -> (64, 16)
  arc A1 (79.375, 23) -> (64, 16) centre (91.4148, -23.8295) ccw projected
  line L5 (79.375, 23) -> (75.1705, 25.8831)
  line L6 (75, 26) -> (79.375, 23) projected
  arc A2 (55.6667, 37) -> (69, 40) centre (60.7425, 45.5702) ccw
  line L7 (69, 40) -> (72, 38)
  arc A3 (72.0011, 38.0008) -> (67.899, 29.0705) centre (72.7517, 32.2487) ccw
  arc A4 (67.899, 29.0705) -> (75, 26) centre (73.7783, 32.9211) ccw
  line L8 (53, 36) -> (55.6667, 37) projected
  line L9 (53, 36) -> (55.6667, 37)
  point P0 (0, 0)
  point P1 (71.9992, 38.0005)
  constraints: 8 end point, 6 point on circle, 3 centre point, 1 collinear, 1 point on line, 1 tangent, 2 other
extrude "Extrusion18" add sketch "Sketch23" along normal blind 1 and the other way blind 21
ref_plane "Work Plane2" through (22, 0, 0) normal (1, 0, 0) x (0, 1, 0)
sketch "Sketch24" plane through (22, 0, 0) normal (1, 0, 0) x (0, 1, 0)
  line L0 (74, 2) -> (64, 2)
  line L1 (74, 2) -> (74, 6)
  line L2 (68, 4) -> (63, 4) projected
  arc A0 (74, 6) -> (64, 2) centre (83, -31) ccw
  point P0 (0, 0)
  constraints: 4 end point, 3 point on circle, 1 centre point, 1 horizontal
emboss "Emboss1" sketch "Sketch24" operation add depth 1 direction (-1, 0, 0) wrap yes faces at (39.3199, 73.9266, 13.3333)
sketch "Sketch25" plane through (22, 0, 0) normal (1, 0, 0) x (0, 1, 0)
  line L0 (74, 18) -> (74, 14)
  line L1 (74, 18) -> (64, 18)
  arc A0 (64, 18) -> (74, 14) centre (83, 51) ccw
  point P0 (0, 0)
  point P1 (68, 16)
  dimension "d94" = 4
  dimension "d96" = 10
  constraints: 4 end point, 3 point on circle, 1 centre point, 1 horizontal, 1 vertical
  measures "d94" distance of L0.start L0.end
  measures "d96" distance of L0.start L1.end
emboss "Emboss2" sketch "Sketch25" operation add depth 1 direction (-1, 0, 0) wrap yes faces at (40.8917, 75.1746, 8.6667)
sketch "Sketch26" plane through (0, 0, -3) normal (0, 0, -1) x (-1, 0, 0)
  point P0 (0, 0)
sketch "Sketch28" plane through (22, 0, 0) normal (1, 0, 0) x (0, 1, 0)
  point P0 (0, 0)
sketch "Sketch29" plane through (22, 0, 0) normal (1, 0, 0) x (0, 1, 0)
  point P0 (0, 0)
ref_plane "Work Plane3" through (0, 42.75, 0) normal (0, 1, 0) x (-1, 0, 0)
sketch "Sketch30" plane through (0, 42.75, 0) normal (0, 1, 0) x (-1, 0, 0)
  circle A0 centre (-106, 6) radius 3
  point P0 (0, 0)
  constraints: 1 centre point
extrude "Extrusion19" add sketch "Sketch30" along normal blind 9 and the other way blind 5
body "Solid1"
